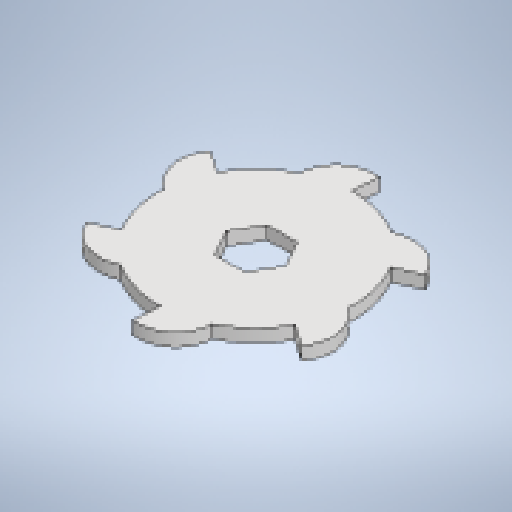
# Autodesk Inventor part: NVPH-202 shredder cutter blade
Saved by Autodesk Inventor 2025.1 (Build 291241020, 241B)
## iProperties
Created: 2024-12-04
Part Number: NVPH-202 shredder cutter blade
Material: Generic
Document SubType Name: Modeling
Designer: DELL
Density: 1 g/cm^3
Appearance: Default
Author: DELL
Autodesk Inventor part; units mm, degrees
ref_plane "YZ Plane" through (0, 0, 0) normal (1, 0, 0) x (0, 1, 0)
ref_plane "XZ Plane" through (0, 0, 0) normal (0, 1, 0) x (-1, 0, 0)
ref_plane "XY Plane" through (0, 0, 0) normal (0, 0, 1) x (1, 0, 0)
sketch "Sketch1" plane through (0, 0, 0) normal (0, 0, 1) x (1, 0, 0)
  line L0 (-11.547, -20) -> (-23.094, 0)
  line L1 (-23.094, 0) -> (-11.547, 20)
  line L2 (-11.547, 20) -> (11.547, 20)
  line L3 (11.547, 20) -> (23.094, 0)
  line L4 (23.094, 0) -> (11.547, -20)
  line L5 (11.547, -20) -> (-11.547, -20)
  circle A0 centre (0, 0) radius 75
  dimension "d0" = 40
  dimension "d2" = 150
  constraints: 12 end point, 1 centre point, 1 coincident, 1 horizontal, 13 other
  measures "d0" distance between parallel lines of L5 L2
  measures "d2" diameter of A0
extrude "Extrusion1" add sketch "Sketch1" along normal blind 10
sketch "Sketch2" plane through (0, 0, 0) normal (0, 0, 1) x (1, 0, 0)
  circle A0 centre (0, 0) radius 75 projected
  line L0 (0, 0) -> (0, 75) construction
  line L1 (0, 95) -> (-15.0761, 73.4691) construction
  line L2 (0, 95) -> (-1.7516, 74.9795)
  circle A1 centre (0, 0) radius 75 projected
  arc A2 (0, 95) -> (-33.7647, 66.9697) centre (-3.8144, 65.2435) ccw
  line L3 (0, 75) -> (0, 95) construction
  point P0 (-1.7516, 74.9795)
  point P1 (-33.7647, 66.9697)
  dimension "d5" = 5
  dimension "d8" = 35
  dimension "d14" = 30
  dimension "d15" = 33
  dimension "d16" = 20
  constraints: 8 end point, 5 point on circle, 2 vertical, 1 centre point, 2 other
  measures "d5" angle of L2 L0
  measures "d8" angle of L0 L1
  measures "d14" radius of A2
  measures "d15" distance of L2.end A2.end
  measures "d16" distance of L0.end L1.start
extrude "Extrusion2" add sketch "Sketch2" along normal blind 10 contours A0 A2 L2
pattern_circular "Circular Pattern1" count 6 over 360 about axis through (0, 0, -10) along (0, 0, 1) of "Extrusion2"
body "Solid1"
